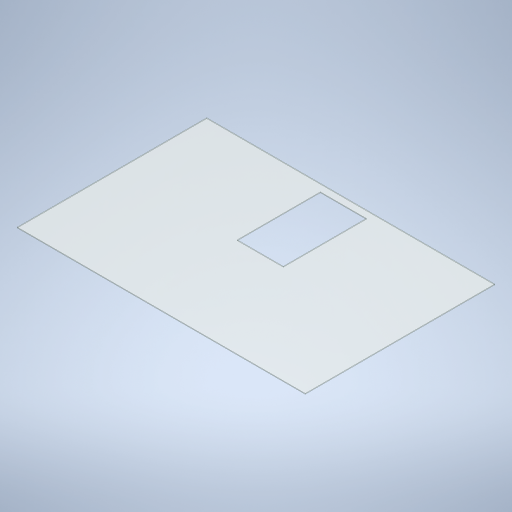
# Autodesk Inventor part: Flooring
Saved by Autodesk Inventor 2024 (Build 280153000, 153)
## iProperties
Created: 2023-05-20
Part Number: Flooring
Material: Wood (Southern Pine)
Document SubType Name: Modeling
Designer: Tom
Density: 7.85 g/cm^3
Appearance: Clear
Author: Tom
Autodesk Inventor part; units mm, degrees
ref_plane "YZ Plane" through (0, 0, 0) normal (1, 0, 0) x (0, 1, 0)
ref_plane "XZ Plane" through (0, 0, 0) normal (0, 1, 0) x (-1, 0, 0)
ref_plane "XY Plane" through (0, 0, 0) normal (0, 0, 1) x (1, 0, 0)
sketch "Sketch1" plane through (0, 0, 0) normal (0, 1, 0) x (-1, 0, 0)
  line L0 (0, 0) -> (7404.1, 0)
  line L1 (7404.1, 0) -> (7404.1, -4871.3898)
  line L2 (7404.1, -4871.3898) -> (0, -4871.3898)
  line L3 (0, -4871.3898) -> (0, 0)
  dimension "d2" = 4871.3898
  dimension "d3" = 7404.1
  constraints: 8 end point, 2 parallel, 1 horizontal, 1 perpendicular
  measures "d2" distance of L2.end L0.start
  measures "d3" distance of L0.start L0.end
extrude "Extrusion1" add sketch "Sketch1" along normal blind 19.05
sketch "Sketch2" plane through (0, 19.05, 0) normal (0, 1, 0) x (1, 0, 0)
  line L0 (-3111.5, 4680.8898) -> (-4292.6, 4680.8898)
  line L1 (-4292.6, 4680.8898) -> (-4292.6, 2547.2898)
  line L2 (-4292.6, 2547.2898) -> (-3111.5, 2547.2898)
  line L3 (-3111.5, 2547.2898) -> (-3111.5, 4680.8898)
  line L4 (0, 0) -> (0, 4871.3898) projected
  line L5 (0, 4871.3898) -> (-7404.1, 4871.3898) projected
  dimension "d6" = 3111.5
  dimension "d7" = 190.5
  dimension "d8" = 1181.1
  dimension "d9" = 2133.6
  constraints: 8 end point, 2 parallel, 1 horizontal, 1 perpendicular
  measures "d6" distance between parallel lines of L4 L3
  measures "d7" distance between parallel lines of L5 L0
  measures "d8" distance between parallel lines of L1 L3
  measures "d9" distance of L0.end L1.end
extrude "Extrusion2" cut sketch "Sketch2" against normal up to surface (19.05 mm away)
body "Solid1"
